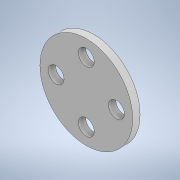
# Autodesk Inventor part: cap
Saved by Autodesk Inventor 2022 (Build 260153000, 153)
## iProperties
Created: 2022-03-08
Part Number: cap
Material: Generic
Document SubType Name: Modeling
Designer: karee
Density: 1 g/cm^3
Appearance: Default
Author: karee
Autodesk Inventor part; units mm, degrees
ref_plane "YZ Plane" through (0, 0, 0) normal (1, 0, 0) x (0, 1, 0)
ref_plane "XZ Plane" through (0, 0, 0) normal (0, 1, 0) x (-1, 0, 0)
ref_plane "XY Plane" through (0, 0, 0) normal (0, 0, 1) x (1, 0, 0)
sketch "Sketch1" plane through (0, 0, 0) normal (0, 0, 1) x (1, 0, 0)
  circle A0 centre (0, 0) radius 3.2004
  line L0 (0, 0) -> (0, 2.0828)
  line L1 (0, 0) -> (2.0828, 0)
  line L2 (0, 0) -> (0, -2.0828)
  line L3 (0, 0) -> (-2.0828, 0)
  circle A1 centre (0, 2.0828) radius 0.5461
  circle A2 centre (2.0828, 0) radius 0.5461
  circle A3 centre (0, -2.0828) radius 0.5461
  circle A4 centre (-2.0828, 0) radius 0.5461
  dimension "d1" = 2.0828
  dimension "d2" = 2.0828
  dimension "d3" = 2.0828
  dimension "d4" = 2.0828
  dimension "d5" = 1.0922
  dimension "d6" = 1.0922
  dimension "d7" = 1.0922
  dimension "d8" = 1.0922
  constraints: 8 end point, 5 centre point, 5 coincident, 2 horizontal, 2 vertical
  measures "d1" distance of L0.start L0.end
  measures "d2" distance of L0.start L1.end
  measures "d3" distance of L0.start L2.end
  measures "d4" distance of L0.start L3.end
  measures "d5" diameter of A1
  measures "d6" diameter of A2
  measures "d7" diameter of A3
  measures "d8" diameter of A4
extrude "Extrusion1" add sketch "Sketch1" along normal blind 0.508
body "Solid1"
